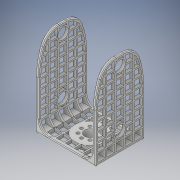
# Autodesk Inventor part: Wheel Case V4
Saved by Autodesk Inventor 2019 (Build 230136000, 136)
## iProperties
Created: 2018-12-01
Part Number: Wheel Case V4
Material: Generic
Document SubType Name: Modeling
Designer: Ashley
Density: 1 g/cm^3
Appearance: Default
Author: Ashley
Autodesk Inventor part; units mm, degrees
ref_plane "YZ Plane" through (0, 0, 0) normal (1, 0, 0) x (0, 1, 0)
ref_plane "XZ Plane" through (0, 0, 0) normal (0, 1, 0) x (-1, 0, 0)
ref_plane "XY Plane" through (0, 0, 0) normal (0, 0, 1) x (1, 0, 0)
sketch "Sketch1" plane through (0, 0, 0) normal (0, 1, 0) x (-1, 0, 0)
  line L0 (40, 32.5) -> (-40, 32.5)
  line L1 (-40, 32.5) -> (-40, -32.5)
  line L2 (-40, -32.5) -> (40, -32.5)
  line L3 (40, -32.5) -> (40, 32.5)
  line L4 (40, 32.5) -> (-40, -32.5) construction
  line L5 (-40, 32.5) -> (40, -32.5) construction
  point P0 (0, 0)
  dimension "d0" = 80
  dimension "d1" = 65
  constraints: 12 end point, 2 midpoint, 2 parallel, 1 horizontal, 1 perpendicular
  measures "d0" distance of L1.end L2.end
  measures "d1" distance of L0.end L1.end
extrude "Top Base Extrusion" add sketch "Sketch1" along normal blind 4
sketch "Sketch2" plane through (0, 4, 0) normal (0, 1, 0) x (1, 0, 0)
  line L0 (-40, -32.5) -> (40, -32.5) construction
  line L1 (40, -32.5) -> (40, 32.5) construction
  line L2 (-40, 32.5) -> (-40, -32.5) construction
  line L3 (-40, 32.5) -> (-36, 32.5)
  line L4 (-36, 32.5) -> (-36, -32.5)
  line L5 (-36, -32.5) -> (-40, -32.5)
  line L6 (-40, -32.5) -> (-40, 32.5)
  line L7 (40, 32.5) -> (36, 32.5)
  line L8 (36, 32.5) -> (36, -32.5)
  line L9 (36, -32.5) -> (40, -32.5)
  line L10 (40, -32.5) -> (40, 32.5)
  point P0 (0, 0)
  dimension "d4" = 4
  dimension "d5" = 4
  constraints: 16 end point, 4 parallel, 2 horizontal, 2 perpendicular, 2 point on line
  measures "d4" distance between parallel lines of L4 L2
  measures "d5" distance between parallel lines of L1 L8
extrude "Side Extrusions" add sketch "Sketch2" along normal blind 110
sketch "Sketch3" plane through (40, 0, 32.5) normal (1, 0, 0) x (0, 0, -1)
  circle A0 centre (32.5, 101.5) radius 7.25
  circle A1 centre (32.5, 26.5) radius 7.25
  line L0 (65, 0) -> (65, 114) construction
  line L1 (0, 114) -> (65, 114) construction
  line L2 (0, 0) -> (0, 114) construction
  line L3 (0, 4) -> (65, 4) construction
  point P0 (32.5, 0)
  dimension "d8" = 14.5
  dimension "d11" = 101.5
  dimension "d43" = 75
  dimension "d44" = 14.5
  dimension "d45" = 65
  dimension "d46" = 32.5
  dimension "d47" = 32.5
  dimension "d48" = 32.5
  dimension "d49" = 12.5
  dimension "d50" = 22.5
  constraints: 2 centre point
  measures "d8" diameter of A0
  measures "d11" distance of point (32.5, 0) A0.centre
  measures "d43" distance of A1.centre A0.centre
  measures "d44" diameter of A1
  measures "d45" distance between parallel lines of L2 L0
  measures "d46" distance from line of L0 A0.centre
  measures "d47" distance from line of L2 A0.centre
  measures "d48" distance from line of L0 A1.centre
  measures "d49" distance from line of A0.centre L1
  measures "d50" distance from line of A1.centre L3
extrude "Wheel Axel Hole" cut sketch "Sketch3" against normal up to surface (80 mm away)
sketch "Sketch4" plane through (0, 0, 0) normal (0, -1, 0) x (1, 0, 0)
  circle A0 centre (0, 0) radius 7.25
  circle A1 centre (0, 0) radius 16
  dimension "d16" = 14.5
  dimension "d17" = 32
  constraints: 2 centre point, 2 coincident
  measures "d16" diameter of A0
  measures "d17" diameter of A1
extrude "Chain Interferance Extrusion" add sketch "Sketch4" along normal blind 6
sketch "Sketch5" plane through (0, 0, 0) normal (0, -1, 0) x (1, 0, 0)
  circle A0 centre (0, 0) radius 7.25 construction
  circle A1 centre (0, 0) radius 7.25
  constraints: 1 centre point, 1 coincident, 1 concentric
extrude "Top Center Bearing Hole" cut sketch "Sketch5" against normal up to surface (4 mm away)
sketch "Sketch7" plane through (0, -6, 0) normal (0, -1, 0) x (1, 0, 0)
  circle A0 centre (0, 0) radius 7.25 construction
  circle A1 centre (0, 11.314) radius 2.05
  circle A2 centre (-8.0002, 8.0002) radius 2.05
  circle A3 centre (-11.314, 0) radius 2.05
  circle A4 centre (-8.0002, -8.0002) radius 2.05
  circle A5 centre (0, -11.314) radius 2.05
  circle A6 centre (8.0002, -8.0002) radius 2.05
  circle A7 centre (11.314, 0) radius 2.05
  circle A8 centre (8.0002, 8.0002) radius 2.05
  dimension "d23" = 4.1
  dimension "d24" = 11.314
  dimension "d27" = 360
  constraints: 8 centre point, 17 other
  measures "d23" diameter of A1
  measures "d24" distance of A0.centre A1.centre
extrude "Sprocket Screws Holes" cut sketch "Sketch7" against normal up to next
sketch "Sketch8" plane through (40, 0, 32.5) normal (1, 0, 0) x (0, 0, -1)
  line L0 (65, 0) -> (65, 114) construction
  line L1 (0, 114) -> (65, 114) construction
  line L2 (0, 0) -> (0, 114) construction
  line L3 (65, 91.5) -> (52.0096, 114)
  line L4 (65, 114) -> (0, 114) construction
  line L5 (65, 91.5) -> (90.9808, 91.5) construction
  line L6 (0, 91.5) -> (34.6363, 91.5) construction
  line L7 (0, 91.5) -> (44.4453, 91.5) construction
  line L8 (0, 91.5) -> (12.9904, 114)
  line L9 (65, 91.5) -> (65, 114)
  line L10 (52.0096, 114) -> (65, 114)
  line L11 (12.9904, 114) -> (0, 114)
  line L12 (0, 91.5) -> (0, 114)
  line L13 (0, 91.5) -> (-31.251, 91.5) construction
  point P0 (32.5, 0)
  dimension "d32" = 120
  dimension "d51" = 120
  constraints: 20 end point, 5 point on line, 3 collinear, 3 horizontal, 1 equal length, 1 perpendicular
  measures "d32" angle of L5 L3
  measures "d51" angle of L13 L8
extrude "Side Corners Cut" cut sketch "Sketch8" against normal up to surface (80 mm away)
fillet "Fillet1" radius 95 4 edges at (38, 91.5, 32.5) (-38, 91.5, 32.5) (38, 91.5, -32.5) (-38, 91.5, -32.5)
fillet "Fillet2" radius 23 4 edges at (38, 114, 19.5096) (38, 114, -19.5096) (-38, 114, -19.5096) (-38, 114, 19.5096)
fillet "Fillet3" radius 3 4 edges at (0, 0, -32.5) (-40, 0, 0) (40, 0, 0) (0, 0, 32.5)
fillet "Fillet4" radius 3 1 edges at (-16, 0, 0)
fillet "Fillet5" radius 1 1 edges at (-16, -6, 0)
sketch "Sketch11" plane through (0, 0, 0) normal (0, -1, 0) x (1, 0, 0)
  line L0 (-37, 29.5) -> (37, 29.5) construction
  line L1 (-37, -29.5) -> (-37, 29.5) construction
  line L2 (37, -29.5) -> (-37, -29.5) construction
  circle A0 centre (0, 0) radius 19 construction
  line L3 (-29, 28) -> (-19, 28)
  line L4 (-19, 28) -> (-19, 18)
  line L5 (-19, 18) -> (-29, 18)
  line L6 (-29, 18) -> (-29, 28)
  line L7 (-17, 28) -> (-7, 28)
  line L8 (-7, 28) -> (-7, 18)
  line L9 (-7, 18) -> (-17, 18)
  line L10 (-17, 18) -> (-17, 28)
  line L11 (-5, 28) -> (5, 28)
  line L12 (5, 28) -> (5, 18)
  line L13 (5, 18) -> (-5, 18)
  line L14 (-5, 18) -> (-5, 28)
  line L15 (7, 28) -> (17, 28)
  line L16 (17, 28) -> (17, 18)
  line L17 (17, 18) -> (7, 18)
  line L18 (7, 18) -> (7, 28)
  line L19 (19, 28) -> (29, 28)
  line L20 (29, 28) -> (29, 18)
  line L21 (29, 18) -> (19, 18)
  line L22 (19, 18) -> (19, 28)
  line L23 (-29, 16.5) -> (-19, 16.5)
  line L24 (-19, 16.5) -> (-19, 6.5)
  line L25 (-19, 6.5) -> (-29, 6.5)
  line L26 (-29, 6.5) -> (-29, 16.5)
  line L27 (-17, 16.5) -> (-7, 16.5)
  line L28 (-7, 16.5) -> (-7, 6.5)
  line L29 (-7, 6.5) -> (-17, 6.5)
  line L30 (-17, 6.5) -> (-17, 16.5)
  line L31 (-5, 16.5) -> (5, 16.5)
  line L32 (5, 16.5) -> (5, 6.5)
  line L33 (5, 6.5) -> (-5, 6.5)
  line L34 (-5, 6.5) -> (-5, 16.5)
  line L35 (7, 16.5) -> (17, 16.5)
  line L36 (17, 16.5) -> (17, 6.5)
  line L37 (17, 6.5) -> (7, 6.5)
  line L38 (7, 6.5) -> (7, 16.5)
  line L39 (19, 16.5) -> (29, 16.5)
  line L40 (29, 16.5) -> (29, 6.5)
  line L41 (29, 6.5) -> (19, 6.5)
  line L42 (19, 6.5) -> (19, 16.5)
  line L43 (-29, 5) -> (-19, 5)
  line L44 (-19, 5) -> (-19, -5)
  line L45 (-19, -5) -> (-29, -5)
  line L46 (-29, -5) -> (-29, 5)
  line L47 (-17, 5) -> (-7, 5)
  line L48 (-7, 5) -> (-7, -5)
  line L49 (-7, -5) -> (-17, -5)
  line L50 (-17, -5) -> (-17, 5)
  line L51 (-5, 5) -> (5, 5)
  line L52 (5, 5) -> (5, -5)
  line L53 (5, -5) -> (-5, -5)
  line L54 (-5, -5) -> (-5, 5)
  line L55 (7, 5) -> (17, 5)
  line L56 (17, 5) -> (17, -5)
  line L57 (17, -5) -> (7, -5)
  line L58 (7, -5) -> (7, 5)
  line L59 (19, 5) -> (29, 5)
  line L60 (29, 5) -> (29, -5)
  line L61 (29, -5) -> (19, -5)
  line L62 (19, -5) -> (19, 5)
  line L63 (-29, -6.5) -> (-19, -6.5)
  line L64 (-19, -6.5) -> (-19, -16.5)
  line L65 (-19, -16.5) -> (-29, -16.5)
  line L66 (-29, -16.5) -> (-29, -6.5)
  line L67 (-17, -6.5) -> (-7, -6.5)
  line L68 (-7, -6.5) -> (-7, -16.5)
  line L69 (-7, -16.5) -> (-17, -16.5)
  line L70 (-17, -16.5) -> (-17, -6.5)
  line L71 (-5, -6.5) -> (5, -6.5)
  line L72 (5, -6.5) -> (5, -16.5)
  line L73 (5, -16.5) -> (-5, -16.5)
  line L74 (-5, -16.5) -> (-5, -6.5)
  line L75 (7, -6.5) -> (17, -6.5)
  line L76 (17, -6.5) -> (17, -16.5)
  line L77 (17, -16.5) -> (7, -16.5)
  line L78 (7, -16.5) -> (7, -6.5)
  line L79 (19, -6.5) -> (29, -6.5)
  line L80 (29, -6.5) -> (29, -16.5)
  line L81 (29, -16.5) -> (19, -16.5)
  line L82 (19, -16.5) -> (19, -6.5)
  line L83 (-29, -18) -> (-19, -18)
  line L84 (-19, -18) -> (-19, -28)
  line L85 (-19, -28) -> (-29, -28)
  line L86 (-29, -28) -> (-29, -18)
  line L87 (-17, -18) -> (-7, -18)
  line L88 (-7, -18) -> (-7, -28)
  line L89 (-7, -28) -> (-17, -28)
  line L90 (-17, -28) -> (-17, -18)
  line L91 (-5, -18) -> (5, -18)
  line L92 (5, -18) -> (5, -28)
  line L93 (5, -28) -> (-5, -28)
  line L94 (-5, -28) -> (-5, -18)
  line L95 (7, -18) -> (17, -18)
  line L96 (17, -18) -> (17, -28)
  line L97 (17, -28) -> (7, -28)
  line L98 (7, -28) -> (7, -18)
  line L99 (19, -18) -> (29, -18)
  line L100 (29, -18) -> (29, -28)
  line L101 (29, -28) -> (19, -28)
  line L102 (19, -28) -> (19, -18)
  line L103 (37, 29.5) -> (37, -29.5) projected
  circle A1 centre (0, 0) radius 7.25 construction
  circle A2 centre (0, 0) radius 20
  point P0 (-17, 10.5357)
  point P1 (-11.3027, 16.5)
  point P2 (-7, 18.735)
  point P3 (-8.7178, 18)
  point P4 (-5, 19.3649)
  point P5 (5, 19.3649)
  point P6 (7, 18.735)
  point P7 (8.7178, 18)
  point P8 (11.3027, 16.5)
  point P9 (17, 10.5357)
  point P10 (19.3649, 5)
  point P11 (19.3649, -5)
  point P12 (17, -10.5357)
  point P13 (11.3027, -16.5)
  point P14 (8.7178, -18)
  point P15 (7, -18.735)
  point P16 (5, -19.3649)
  point P17 (-5, -19.3649)
  point P18 (-8.7178, -18)
  point P19 (-7, -18.735)
  point P20 (-11.3027, -16.5)
  point P21 (-17, -10.5357)
  point P22 (-19.3649, -5)
  point P23 (-19.3649, 5)
  dimension "d309" = 40
  dimension "d259" = 10
  dimension "d260" = 10
  dimension "d262" = 1.5
  dimension "d263" = 8
  dimension "d266" = 12
  dimension "d269" = 11.5
  dimension "d272" = 1.5
  dimension "d307" = 8
  dimension "d308" = 38
  constraints: 200 end point, 23 point on line, 2 horizontal, 2 parallel, 1 coincident, 1 perpendicular, 1 vertical, 218 other
  measures "d259" distance of L3.start L3.end
  measures "d260" distance of L3.end L4.end
  measures "d262" distance between parallel lines of L0 L3
  measures "d263" distance between parallel lines of L1 L6
  measures "d266" distance of L3.start L7.start
  measures "d269" distance of L3.start L23.start
  measures "d272" distance between parallel lines of L2 L85
  measures "d307" distance between parallel lines of L103 L20
  measures "d308" diameter of A0
fillet "Fillet8" radius 14 2 edges at (-36, 4, 0) (36, 4, 0)
fillet "Fillet9" radius 1 38 edges at (36, 42.0224, 32.5) (36, 82.7695, 31.0162) (36, 109.8726, 18.1832) (36, 114, 0) (36, 109.8726, -18.1832) (36, 82.7695, -31.0162) (36, 42.0224, -32.5) (31.8995, 8.1005, -32.5) (0, 4, -32.5) (-31.8995, 8.1005, -32.5) (-36, 42.0224, -32.5) (-36, 82.7695, -31.0162) (-36, 109.8726, -18.1832) (-36, 114, 0) (-36, 109.8726, 18.1832) (-36, 82.7695, 31.0162) (-36, 42.0224, 32.5) (-31.8995, 8.1005, 32.5) (0, 4, 32.5) (31.8995, 8.1005, 32.5) (40, 82.7695, 31.0162) (40, 109.8726, 18.1832) (40, 114, 0) (40, 109.8726, -18.1832) (40, 82.7695, -31.0162) (40, 34.5224, -32.5) (39.1213, 0.8787, -31.6213) (39.1213, 0.8787, 31.6213) (40, 34.5224, 32.5) (-40, 82.7695, 31.0162) (-40, 109.8726, 18.1832) (-40, 114, 0) (-40, 109.8726, -18.1832) (-40, 82.7695, -31.0162) (-40, 34.5224, -32.5) (-39.1213, 0.8787, -31.6213) (-39.1213, 0.8787, 31.6213) (-40, 34.5224, 32.5)
sketch "Sketch12" plane through (40, 3, -31.5) normal (1, 0, 0) x (0, 0, -1)
  circle A0 centre (-31.5, 98.5) radius 7.25 construction
  circle A1 centre (-31.5, 23.5) radius 7.25 construction
  line L0 (0, 63.0448) -> (0, 0) construction
  arc A2 (0, 63.0448) -> (-5.8268, 95.6252) centre (-94, 63.0448) ccw construction
  arc A3 (-5.8268, 95.6252) -> (-26.4631, 110) centre (-26.4631, 88) ccw construction
  arc A4 (-36.5369, 110) -> (-57.1732, 95.6252) centre (-36.5369, 88) ccw construction
  arc A5 (-57.1732, 95.6252) -> (-63, 63.0448) centre (31, 63.0448) ccw construction
  line L1 (-63, 0) -> (-63, 63.0448) construction
  line L2 (0, 0) -> (-63, 0) construction
  line L3 (-61.1, 12) -> (-51.1, 12)
  line L4 (-51.1, 12) -> (-51.1, 2)
  line L5 (-51.1, 2) -> (-61.1, 2)
  line L6 (-61.1, 2) -> (-61.1, 12)
  line L7 (-61.1, 24) -> (-51.1, 24)
  line L8 (-51.1, 24) -> (-51.1, 14)
  line L9 (-51.1, 14) -> (-61.1, 14)
  line L10 (-61.1, 14) -> (-61.1, 24)
  line L11 (-61.1, 36) -> (-51.1, 36)
  line L12 (-51.1, 36) -> (-51.1, 26)
  line L13 (-51.1, 26) -> (-61.1, 26)
  line L14 (-61.1, 26) -> (-61.1, 36)
  line L15 (-61.1, 48) -> (-51.1, 48)
  line L16 (-51.1, 48) -> (-51.1, 38)
  line L17 (-51.1, 38) -> (-61.1, 38)
  line L18 (-61.1, 38) -> (-61.1, 48)
  line L19 (-61.1, 60) -> (-51.1, 60)
  line L20 (-51.1, 60) -> (-51.1, 50)
  line L21 (-51.1, 50) -> (-61.1, 50)
  line L22 (-61.1, 50) -> (-61.1, 60)
  line L23 (-61.1, 72) -> (-51.1, 72)
  line L24 (-51.1, 72) -> (-51.1, 62)
  line L25 (-51.1, 62) -> (-61.1, 62)
  line L26 (-61.1, 62) -> (-61.1, 72)
  line L27 (-61.1, 84) -> (-51.1, 84)
  line L28 (-51.1, 84) -> (-51.1, 74)
  line L29 (-51.1, 74) -> (-61.1, 74)
  line L30 (-61.1, 74) -> (-61.1, 84)
  line L31 (-61.1, 96) -> (-51.1, 96)
  line L32 (-51.1, 96) -> (-51.1, 86)
  line L33 (-51.1, 86) -> (-61.1, 86)
  line L34 (-61.1, 86) -> (-61.1, 96)
  line L35 (-61.1, 108) -> (-51.1, 108)
  line L36 (-51.1, 108) -> (-51.1, 98)
  line L37 (-51.1, 98) -> (-61.1, 98)
  line L38 (-61.1, 98) -> (-61.1, 108)
  line L39 (-48.8, 12) -> (-38.8, 12)
  line L40 (-38.8, 12) -> (-38.8, 2)
  line L41 (-38.8, 2) -> (-48.8, 2)
  line L42 (-48.8, 2) -> (-48.8, 12)
  line L43 (-48.8, 24) -> (-38.8, 24)
  line L44 (-38.8, 24) -> (-38.8, 14)
  line L45 (-38.8, 14) -> (-48.8, 14)
  line L46 (-48.8, 14) -> (-48.8, 24)
  line L47 (-48.8, 36) -> (-38.8, 36)
  line L48 (-38.8, 36) -> (-38.8, 26)
  line L49 (-38.8, 26) -> (-48.8, 26)
  line L50 (-48.8, 26) -> (-48.8, 36)
  line L51 (-48.8, 48) -> (-38.8, 48)
  line L52 (-38.8, 48) -> (-38.8, 38)
  line L53 (-38.8, 38) -> (-48.8, 38)
  line L54 (-48.8, 38) -> (-48.8, 48)
  line L55 (-48.8, 60) -> (-38.8, 60)
  line L56 (-38.8, 60) -> (-38.8, 50)
  line L57 (-38.8, 50) -> (-48.8, 50)
  line L58 (-48.8, 50) -> (-48.8, 60)
  line L59 (-48.8, 72) -> (-38.8, 72)
  line L60 (-38.8, 72) -> (-38.8, 62)
  line L61 (-38.8, 62) -> (-48.8, 62)
  line L62 (-48.8, 62) -> (-48.8, 72)
  line L63 (-48.8, 84) -> (-38.8, 84)
  line L64 (-38.8, 84) -> (-38.8, 74)
  line L65 (-38.8, 74) -> (-48.8, 74)
  line L66 (-48.8, 74) -> (-48.8, 84)
  line L67 (-48.8, 96) -> (-38.8, 96)
  line L68 (-38.8, 96) -> (-38.8, 86)
  line L69 (-38.8, 86) -> (-48.8, 86)
  line L70 (-48.8, 86) -> (-48.8, 96)
  line L71 (-48.8, 108) -> (-38.8, 108)
  line L72 (-38.8, 108) -> (-38.8, 98)
  line L73 (-38.8, 98) -> (-48.8, 98)
  line L74 (-48.8, 98) -> (-48.8, 108)
  line L75 (-36.5, 12) -> (-26.5, 12)
  line L76 (-26.5, 12) -> (-26.5, 2)
  line L77 (-26.5, 2) -> (-36.5, 2)
  line L78 (-36.5, 2) -> (-36.5, 12)
  line L79 (-36.5, 24) -> (-26.5, 24)
  line L80 (-26.5, 24) -> (-26.5, 14)
  line L81 (-26.5, 14) -> (-36.5, 14)
  line L82 (-36.5, 14) -> (-36.5, 24)
  line L83 (-36.5, 36) -> (-26.5, 36)
  line L84 (-26.5, 36) -> (-26.5, 26)
  line L85 (-26.5, 26) -> (-36.5, 26)
  line L86 (-36.5, 26) -> (-36.5, 36)
  line L87 (-36.5, 48) -> (-26.5, 48)
  line L88 (-26.5, 48) -> (-26.5, 38)
  line L89 (-26.5, 38) -> (-36.5, 38)
  line L90 (-36.5, 38) -> (-36.5, 48)
  line L91 (-36.5, 60) -> (-26.5, 60)
  line L92 (-26.5, 60) -> (-26.5, 50)
  line L93 (-26.5, 50) -> (-36.5, 50)
  line L94 (-36.5, 50) -> (-36.5, 60)
  line L95 (-36.5, 72) -> (-26.5, 72)
  line L96 (-26.5, 72) -> (-26.5, 62)
  line L97 (-26.5, 62) -> (-36.5, 62)
  line L98 (-36.5, 62) -> (-36.5, 72)
  line L99 (-36.5, 84) -> (-26.5, 84)
  line L100 (-26.5, 84) -> (-26.5, 74)
  line L101 (-26.5, 74) -> (-36.5, 74)
  line L102 (-36.5, 74) -> (-36.5, 84)
  line L103 (-36.5, 96) -> (-26.5, 96)
  line L104 (-26.5, 96) -> (-26.5, 86)
  line L105 (-26.5, 86) -> (-36.5, 86)
  line L106 (-36.5, 86) -> (-36.5, 96)
  line L107 (-36.5, 108) -> (-26.5, 108)
  line L108 (-26.5, 108) -> (-26.5, 98)
  line L109 (-26.5, 98) -> (-36.5, 98)
  line L110 (-36.5, 98) -> (-36.5, 108)
  line L111 (-24.2, 12) -> (-14.2, 12)
  line L112 (-14.2, 12) -> (-14.2, 2)
  line L113 (-14.2, 2) -> (-24.2, 2)
  line L114 (-24.2, 2) -> (-24.2, 12)
  line L115 (-24.2, 24) -> (-14.2, 24)
  line L116 (-14.2, 24) -> (-14.2, 14)
  line L117 (-14.2, 14) -> (-24.2, 14)
  line L118 (-24.2, 14) -> (-24.2, 24)
  line L119 (-24.2, 36) -> (-14.2, 36)
  line L120 (-14.2, 36) -> (-14.2, 26)
  line L121 (-14.2, 26) -> (-24.2, 26)
  line L122 (-24.2, 26) -> (-24.2, 36)
  line L123 (-24.2, 48) -> (-14.2, 48)
  line L124 (-14.2, 48) -> (-14.2, 38)
  line L125 (-14.2, 38) -> (-24.2, 38)
  line L126 (-24.2, 38) -> (-24.2, 48)
  line L127 (-24.2, 60) -> (-14.2, 60)
  line L128 (-14.2, 60) -> (-14.2, 50)
  line L129 (-14.2, 50) -> (-24.2, 50)
  line L130 (-24.2, 50) -> (-24.2, 60)
  line L131 (-24.2, 72) -> (-14.2, 72)
  line L132 (-14.2, 72) -> (-14.2, 62)
  line L133 (-14.2, 62) -> (-24.2, 62)
  line L134 (-24.2, 62) -> (-24.2, 72)
  line L135 (-24.2, 84) -> (-14.2, 84)
  line L136 (-14.2, 84) -> (-14.2, 74)
  line L137 (-14.2, 74) -> (-24.2, 74)
  line L138 (-24.2, 74) -> (-24.2, 84)
  line L139 (-24.2, 96) -> (-14.2, 96)
  line L140 (-14.2, 96) -> (-14.2, 86)
  line L141 (-14.2, 86) -> (-24.2, 86)
  line L142 (-24.2, 86) -> (-24.2, 96)
  line L143 (-24.2, 108) -> (-14.2, 108)
  line L144 (-14.2, 108) -> (-14.2, 98)
  line L145 (-14.2, 98) -> (-24.2, 98)
  line L146 (-24.2, 98) -> (-24.2, 108)
  line L147 (-11.9, 12) -> (-1.9, 12)
  line L148 (-1.9, 12) -> (-1.9, 2)
  line L149 (-1.9, 2) -> (-11.9, 2)
  line L150 (-11.9, 2) -> (-11.9, 12)
  line L151 (-11.9, 24) -> (-1.9, 24)
  line L152 (-1.9, 24) -> (-1.9, 14)
  line L153 (-1.9, 14) -> (-11.9, 14)
  line L154 (-11.9, 14) -> (-11.9, 24)
  line L155 (-11.9, 36) -> (-1.9, 36)
  line L156 (-1.9, 36) -> (-1.9, 26)
  line L157 (-1.9, 26) -> (-11.9, 26)
  line L158 (-11.9, 26) -> (-11.9, 36)
  line L159 (-11.9, 48) -> (-1.9, 48)
  line L160 (-1.9, 48) -> (-1.9, 38)
  line L161 (-1.9, 38) -> (-11.9, 38)
  line L162 (-11.9, 38) -> (-11.9, 48)
  line L163 (-11.9, 60) -> (-1.9, 60)
  line L164 (-1.9, 60) -> (-1.9, 50)
  line L165 (-1.9, 50) -> (-11.9, 50)
  line L166 (-11.9, 50) -> (-11.9, 60)
  line L167 (-11.9, 72) -> (-1.9, 72)
  line L168 (-1.9, 72) -> (-1.9, 62)
  line L169 (-1.9, 62) -> (-11.9, 62)
  line L170 (-11.9, 62) -> (-11.9, 72)
  line L171 (-11.9, 84) -> (-1.9, 84)
  line L172 (-1.9, 84) -> (-1.9, 74)
  line L173 (-1.9, 74) -> (-11.9, 74)
  line L174 (-11.9, 74) -> (-11.9, 84)
  line L175 (-11.9, 96) -> (-1.9, 96)
  line L176 (-1.9, 96) -> (-1.9, 86)
  line L177 (-1.9, 86) -> (-11.9, 86)
  line L178 (-11.9, 86) -> (-11.9, 96)
  line L179 (-11.9, 108) -> (-1.9, 108)
  line L180 (-1.9, 108) -> (-1.9, 98)
  line L181 (-1.9, 98) -> (-11.9, 98)
  line L182 (-11.9, 98) -> (-11.9, 108)
  arc A6 (-57.1732, 95.6252) -> (-63, 63.0448) centre (31, 63.0448) ccw construction
  arc A7 (0, 63.0448) -> (-5.8268, 95.6252) centre (-94, 63.0448) ccw construction
  arc A8 (-5.8268, 95.6252) -> (-26.4631, 110) centre (-26.4631, 88) ccw construction
  line L183 (-26.4631, 110) -> (-36.5369, 110) construction
  arc A9 (-36.5369, 110) -> (-57.1732, 95.6252) centre (-36.5369, 88) ccw construction
  line L184 (-57.1732, 95.6252) -> (-58.1113, 95.9718) construction
  line L185 (-26.4631, 110) -> (-26.4631, 111) construction
  line L186 (0, 15) -> (0, 63.0448) construction
  circle A10 centre (-31.5, 23.5) radius 9
  arc A11 (-55.391, 94.9667) -> (-61.0769, 60.9831) centre (31, 63.0448) ccw
  arc A12 (-36.5369, 108.1) -> (-55.391, 94.9667) centre (-36.5369, 88) ccw
  arc A13 (-1.9838, 59.1159) -> (-7.609, 94.9667) centre (-94, 63.0448) ccw
  arc A14 (-7.609, 94.9667) -> (-26.4631, 108.1) centre (-26.4631, 88) ccw
  line L187 (-26.4631, 108.1) -> (-36.5369, 108.1)
  circle A15 centre (-31.5, 98.5) radius 9
  point P0 (-31.5, -3)
  point P1 (-40.4861, 98)
  point P2 (-36.5, 30.9833)
  point P3 (-26.5, 30.9833)
  point P4 (-24.2, 28.764)
  point P5 (-22.8542, 26)
  point P6 (-22.5139, 24)
  point P7 (-24.2, 18.236)
  point P8 (-26.5, 16.0167)
  point P9 (-36.5, 16.0167)
  point P10 (-38.8, 18.236)
  point P11 (-40.4861, 24)
  point P12 (-40.1458, 26)
  point P13 (-38.8, 28.764)
  point P14 (-24.2, 107.9722)
  point P15 (-14.2, 103.9257)
  point P16 (-11.9, 101.8538)
  point P17 (-9.0272, 98)
  point P18 (-8.0237, 96)
  point P19 (-4.8066, 86)
  point P20 (-4.3156, 84)
  point P21 (-2.5539, 74)
  point P22 (-2.3364, 72)
  point P23 (-1.9, 63.0448)
  point P24 (-38.8, 107.9722)
  point P25 (-48.8, 103.9257)
  point P26 (-51.1, 101.8538)
  point P27 (-53.9728, 98)
  point P28 (-54.9763, 96)
  point P29 (-58.1934, 86)
  point P30 (-58.6844, 84)
  point P31 (-60.4461, 74)
  point P32 (-60.6636, 72)
  point P33 (-61.1, 63.0448)
  point P34 (-26.5, 105.9833)
  point P35 (-24.2, 103.764)
  point P36 (-22.5139, 98)
  point P37 (-22.8542, 96)
  point P38 (-24.2, 93.236)
  point P39 (-38.8, 93.236)
  point P40 (-40.4861, 98)
  point P41 (-36.5, 105.9833)
  point P42 (-36.5, 91.0167)
  point P43 (-26.5, 91.0167)
  point P44 (-38.8, 103.764)
  point P45 (-40.4861, 98)
  point P46 (-40.1458, 96)
  dimension "d298" = 18
  dimension "d304" = 18
  dimension "d277" = 10
  dimension "d278" = 10
  dimension "d279" = 1.9
  dimension "d280" = 2
  dimension "d283" = 12
  dimension "d286" = 12.3
  dimension "d289" = 1.9
  dimension "d290" = 94
  dimension "d292" = 94
  dimension "d293" = 22
  dimension "d294" = 22
  dimension "d300" = 92.1
  dimension "d301" = 20.1
  dimension "d302" = 92.1
  dimension "d303" = 20.1
  constraints: 362 end point, 44 point on line, 28 point on circle, 8 coincident, 4 centre point, 3 horizontal, 3 parallel, 1 perpendicular, 1 vertical, 379 other
  measures "d277" distance between parallel lines of L4 L6
  measures "d278" distance between parallel lines of L5 L3
  measures "d279" distance between parallel lines of L1 L6
  measures "d280" distance between parallel lines of L2 L5
  measures "d283" distance of L3.end L7.end
  measures "d286" distance of L3.end L39.end
  measures "d289" distance between parallel lines of L0 L148
  measures "d290" radius of A5
  measures "d292" radius of A2
  measures "d293" radius of A4
  measures "d294" radius of A3
  measures "d300" radius of A11
  measures "d301" radius of A12
  measures "d302" radius of A13
  measures "d303" radius of A14
extrude "Extrusion11" cut sketch "Sketch12" against normal up to surface (80 mm away) contours L3 L4 L5 L6 | L7 L8 L9 L10 | L11 L12 L13 L14 | L15 L16 L17 L18 | L19 L20 L21 L22 | L163 L164 L165 L166 | A13 L169 L170 L167 | A13 L173 L174 L171 | A14 A13 L177 L178 L175 | A14 L181 L182 | A12 L72 A15 L73 L74 | A12 L36 L37 | A11 A12 L31 L32 L33 | A11 L27 L28 L29 | L23 L24 L25 A11 | A11 L25 L26 | A15 L72 L73 | A15 L68 L69 L70 L67 | L110 L107 L108 A15 | A14 L144 L145 A15 L146 | A15 L104 L105 L106 | A15 L139 L140 L141 L142 | L168 L169 A13 | L39 L40 L41 L42 | L43 A10 L44 L45 L46 | L49 L50 L47 L48 A10 | A10 L80 L81 L82 | L86 L83 L84 A10 | A10 L115 L116 L117 L118 | L122 L119 L120 L121 A10 | L51 L52 L53 L54 | L55 L56 L57 L58 | L59 L60 L61 L62 | L63 L64 L65 L66 | L75 L76 L77 L78 | L87 L88 L89 L90 | L91 L92 L93 L94 | L95 L96 L97 L98 | L99 L100 L101 L102 | L111 L112 L113 L114 | L123 L124 L125 L126 | L127 L128 L129 L130 | L131 L132 L133 L134 | L135 L136 L137 L138 | L147 L148 L149 L150 | L151 L152 L153 L154 | L155 L156 L157 L158 | L159 L160 L161 L162
extrude "Extrusion12" cut sketch "Sketch11" against normal through all contours L3 L4 L5 L6 | L7 L8 A2 L9 L10 | L14 L11 L12 A2 | A2 L30 L27 | A2 L17 L18 | L18 L15 L16 L17 A2 | A2 L45 L46 L43 | L35 L36 A2 | A2 L69 L70 | L59 L60 L61 A2 | A2 L88 L89 L90 L87 | A2 L92 L93 L94 | L76 L77 A2 | A2 L95 L96 L97 L98 | L19 L20 L21 L22 | L23 L24 L25 L26 | L39 L40 L41 L42 | L63 L64 L65 L66 | L79 L80 L81 L82 | L83 L84 L85 L86 | L99 L100 L101 L102
body "Solid1"
